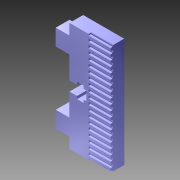
# Autodesk Inventor part: brida correas eje y
Saved by Autodesk Inventor 2012 SP2 (Build 160219200, 219)
## iProperties
Created: 2014-07-08
Part Number: brida correas eje y
Material: Default
Document SubType Name: Modeling
Designer: Principal
Density: 1 g/cm^3
Author: Principal
Autodesk Inventor part; units mm, degrees
ref_plane "YZ Plane" through (0, 0, 0) normal (1, 0, 0) x (0, 1, 0)
ref_plane "XZ Plane" through (0, 0, 0) normal (0, 1, 0) x (-1, 0, 0)
ref_plane "XY Plane" through (0, 0, 0) normal (0, 0, 1) x (1, 0, 0)
sketch "Boceto1" plane through (0, 0, 0) normal (0, 0, 1) x (1, 0, 0)
  line L0 (0, 0) -> (15, 0)
  line L1 (15, 0) -> (15, -5)
  line L2 (15, -5) -> (0, -5)
  line L3 (0, -5) -> (0, 0)
  constraints: 8 end point
extrude "Extrusión1" add sketch "Boceto1" along normal blind 40
sketch "Boceto2" plane through (0, 0, 0) normal (0, 1, 0) x (1, 0, 0)
  line L0 (0, -40) -> (15, -40) projected
  line L1 (6.174, -21.75) -> (6.174, -18.25)
  line L2 (2.774, -22.75) -> (5.174, -22.75)
  line L3 (5.174, -17.25) -> (2.774, -17.25)
  line L4 (6.174, -18.25) -> (5.174, -18.25)
  line L5 (2.774, -18.25) -> (0, -18.25)
  line L6 (2.774, -17.25) -> (2.774, -18.25)
  line L7 (2.774, -21.75) -> (2.774, -22.75)
  line L8 (5.174, -22.75) -> (5.174, -21.75)
  line L9 (5.174, -18.25) -> (5.174, -17.25)
  line L10 (0, -21.75) -> (2.774, -21.75)
  line L11 (5.174, -21.75) -> (6.174, -21.75)
  line L12 (0, -10) -> (-5, -10)
  line L13 (-5, -10) -> (-5, -4)
  line L14 (-5, -4) -> (0, -4)
  line L15 (0, -4) -> (0, -10)
  line L16 (0, -36) -> (-5, -36)
  line L17 (-5, -36) -> (-5, -30)
  line L18 (-5, -30) -> (0, -30)
  line L19 (0, -30) -> (0, -36)
  line L20 (0, 0) -> (0, -40) projected
  dimension "d7" = 3.5
  dimension "d8" = 2.4
  dimension "d12" = 18.25
  dimension "d14" = 6
  dimension "d15" = 5
  dimension "d16" = 5
  dimension "d17" = 6
  dimension "d18" = 4
  dimension "d19" = 20
  constraints: 38 end point, 2 point on line
  measures "d7" distance of L1.end L1.start
  measures "d8" distance of L3.end L3.start
  measures "d12" distance from line of L0 L1.start
  measures "d14" distance between parallel lines of L18 L16
  measures "d15" distance between parallel lines of L19 L17
  measures "d16" distance between parallel lines of L15 L13
  measures "d17" distance between parallel lines of L12 L14
  measures "d18" distance between parallel lines of L0 L16
  measures "d19" distance between parallel lines of L12 L18
extrude "Extrusión3" cut sketch "Boceto2" against normal through all
sketch "Boceto3" plane through (0, 0, 0) normal (0, 1, 0) x (1, 0, 0)
  line L0 (2.774, -21.75) -> (0, -21.75) projected
  line L1 (0, -18.25) -> (2.774, -18.25) projected
  line L2 (-5, -10) -> (-5, -4)
  line L3 (-5, -36) -> (-5, -30)
  line L4 (-5, -36) -> (0, -36)
  line L5 (-5, -30) -> (0, -30)
  line L6 (-5, -4) -> (0, -4)
  line L7 (-5, -10) -> (0, -10)
  line L8 (0, -4) -> (0, -10)
  line L9 (0, -30) -> (0, -36)
  constraints: 18 end point
extrude "Extrusión4" add sketch "Boceto3" against normal blind 5
sketch "Boceto4" plane through (15, -5, 0) normal (1, 0, 0) x (0, 0, -1)
  arc A0 (-37.4947, 0.496) -> (-38.4947, 0.496) centre (-37.9947, 0.496) ccw
  line L0 (-38.4947, 0.496) -> (-38.4947, -0.004)
  line L1 (-37.4947, 0.496) -> (-37.4947, -0.004)
  line L2 (-39.4947, 0.496) -> (-39.4947, -0.004)
  arc A1 (-39.4947, 0.496) -> (-39.9947, 0.996) centre (-39.9947, 0.496) ccw
  arc A2 (-35.9947, 0.996) -> (-36.4947, 0.496) centre (-35.9947, 0.496) ccw
  line L3 (-36.4947, -0.004) -> (-36.4947, 0.496)
  arc A3 (-33.4947, 0.496) -> (-34.4947, 0.496) centre (-33.9947, 0.496) ccw
  line L4 (-34.4947, 0.496) -> (-34.4947, -0.004)
  line L5 (-33.4947, 0.496) -> (-33.4947, -0.004)
  line L6 (-35.4947, 0.496) -> (-35.4947, -0.004)
  arc A4 (-35.4947, 0.496) -> (-35.9947, 0.996) centre (-35.9947, 0.496) ccw
  arc A5 (-31.9947, 0.996) -> (-32.4947, 0.496) centre (-31.9947, 0.496) ccw
  line L7 (-32.4947, -0.004) -> (-32.4947, 0.496)
  arc A6 (-29.4947, 0.496) -> (-30.4947, 0.496) centre (-29.9947, 0.496) ccw
  line L8 (-30.4947, 0.496) -> (-30.4947, -0.004)
  line L9 (-29.4947, 0.496) -> (-29.4947, -0.004)
  line L10 (-31.4947, 0.496) -> (-31.4947, -0.004)
  arc A7 (-31.4947, 0.496) -> (-31.9947, 0.996) centre (-31.9947, 0.496) ccw
  arc A8 (-27.9947, 0.996) -> (-28.4947, 0.496) centre (-27.9947, 0.496) ccw
  line L11 (-28.4947, -0.004) -> (-28.4947, 0.496)
  line L12 (-26.4947, 0.496) -> (-26.4947, -0.004)
  line L13 (-25.4947, 0.496) -> (-25.4947, -0.004)
  line L14 (-27.4947, 0.496) -> (-27.4947, -0.004)
  line L15 (-24.4947, -0.004) -> (-24.4947, 0.496)
  arc A9 (-23.9947, 0.996) -> (-24.4947, 0.496) centre (-23.9947, 0.496) ccw
  arc A10 (-25.4947, 0.496) -> (-26.4947, 0.496) centre (-25.9947, 0.496) ccw
  arc A11 (-27.4947, 0.496) -> (-27.9947, 0.996) centre (-27.9947, 0.496) ccw
  arc A12 (-21.4947, 0.496) -> (-22.4947, 0.496) centre (-21.9947, 0.496) ccw
  line L16 (-22.4947, 0.496) -> (-22.4947, -0.004)
  line L17 (-21.4947, 0.496) -> (-21.4947, -0.004)
  line L18 (-23.4947, 0.496) -> (-23.4947, -0.004)
  arc A13 (-23.4947, 0.496) -> (-23.9947, 0.996) centre (-23.9947, 0.496) ccw
  arc A14 (-19.9947, 0.996) -> (-20.4947, 0.496) centre (-19.9947, 0.496) ccw
  line L19 (-20.4947, -0.004) -> (-20.4947, 0.496)
  line L20 (-18.4947, 0.496) -> (-18.4947, -0.004)
  line L21 (-17.4947, 0.496) -> (-17.4947, -0.004)
  line L22 (-19.4947, 0.496) -> (-19.4947, -0.004)
  line L23 (-16.4947, -0.004) -> (-16.4947, 0.496)
  arc A15 (-15.9947, 0.996) -> (-16.4947, 0.496) centre (-15.9947, 0.496) ccw
  arc A16 (-17.4947, 0.496) -> (-18.4947, 0.496) centre (-17.9947, 0.496) ccw
  arc A17 (-19.4947, 0.496) -> (-19.9947, 0.996) centre (-19.9947, 0.496) ccw
  arc A18 (-15.4947, 0.496) -> (-15.9947, 0.996) centre (-15.9947, 0.496) ccw
  line L24 (-14.4947, 0.496) -> (-14.4947, -0.004)
  arc A19 (-13.4947, 0.496) -> (-14.4947, 0.496) centre (-13.9947, 0.496) ccw
  line L25 (-13.4947, 0.496) -> (-13.4947, -0.004)
  line L26 (-12.4947, -0.004) -> (-12.4947, 0.496)
  arc A20 (-11.9947, 0.996) -> (-12.4947, 0.496) centre (-11.9947, 0.496) ccw
  arc A21 (-11.4947, 0.496) -> (-11.9947, 0.996) centre (-11.9947, 0.496) ccw
  line L27 (-11.4947, 0.496) -> (-11.4947, -0.004)
  line L28 (-15.4947, 0.496) -> (-15.4947, -0.004)
  line L29 (-10.4947, 0.496) -> (-10.4947, -0.004)
  arc A22 (-9.4947, 0.496) -> (-10.4947, 0.496) centre (-9.9947, 0.496) ccw
  line L30 (-9.4947, 0.496) -> (-9.4947, -0.004)
  line L31 (-8.4947, -0.004) -> (-8.4947, 0.496)
  arc A23 (-7.9947, 0.996) -> (-8.4947, 0.496) centre (-7.9947, 0.496) ccw
  arc A24 (0.0053, 0.996) -> (-0.4947, 0.496) centre (0.0053, 0.496) ccw
  line L32 (-0.4947, -0.004) -> (-0.4947, 0.496)
  arc A25 (-5.4947, 0.496) -> (-6.4947, 0.496) centre (-5.9947, 0.496) ccw
  line L33 (-6.4947, 0.496) -> (-6.4947, -0.004)
  line L34 (-7.4947, 0.496) -> (-7.4947, -0.004)
  arc A26 (-7.4947, 0.496) -> (-7.9947, 0.996) centre (-7.9947, 0.496) ccw
  line L35 (-5.4947, 0.496) -> (-5.4947, -0.004)
  line L36 (-4.4947, -0.004) -> (-4.4947, 0.496)
  arc A27 (-3.9947, 0.996) -> (-4.4947, 0.496) centre (-3.9947, 0.496) ccw
  arc A28 (-3.4947, 0.496) -> (-3.9947, 0.996) centre (-3.9947, 0.496) ccw
  line L37 (-3.4947, 0.496) -> (-3.4947, -0.004)
  line L38 (-2.4947, 0.496) -> (-2.4947, -0.004)
  arc A29 (-1.4947, 0.496) -> (-2.4947, 0.496) centre (-1.9947, 0.496) ccw
  line L39 (-1.4947, 0.496) -> (-1.4947, -0.004)
  line L40 (-0.4947, -0.004) -> (0.0053, -0.004)
  line L41 (-2.4947, -0.004) -> (-1.4947, -0.004)
  line L42 (-4.4947, -0.004) -> (-3.4947, -0.004)
  line L43 (-6.4947, -0.004) -> (-5.4947, -0.004)
  line L44 (-8.4947, -0.004) -> (-7.4947, -0.004)
  line L45 (-10.4947, -0.004) -> (-9.4947, -0.004)
  line L46 (-12.4947, -0.004) -> (-11.4947, -0.004)
  line L47 (-14.4947, -0.004) -> (-13.4947, -0.004)
  line L48 (-16.4947, -0.004) -> (-15.4947, -0.004)
  line L49 (-18.4947, -0.004) -> (-17.4947, -0.004)
  line L50 (-24.4947, -0.004) -> (-23.4947, -0.004)
  line L51 (-22.4947, -0.004) -> (-21.4947, -0.004)
  line L52 (-20.4947, -0.004) -> (-19.4947, -0.004)
  line L53 (-26.4947, -0.004) -> (-25.4947, -0.004)
  line L54 (-28.4947, -0.004) -> (-27.4947, -0.004)
  line L55 (-30.4947, -0.004) -> (-29.4947, -0.004)
  line L56 (-32.4947, -0.004) -> (-31.4947, -0.004)
  line L57 (-34.4947, -0.004) -> (-33.4947, -0.004)
  line L58 (-36.4947, -0.004) -> (-35.4947, -0.004)
  line L59 (-39.9947, -0.004) -> (-39.4947, -0.004)
  line L60 (-38.4947, -0.004) -> (-37.4947, -0.004)
  line L61 (0.0053, -0.004) -> (0.0053, 0.996)
  line L62 (-39.9947, -0.004) -> (-40.0154, -0.004)
  line L63 (-40.0154, -0.004) -> (-40.0154, 0.996)
  line L64 (-40.0154, 0.996) -> (-39.9947, 0.996)
  point P0 (-32.9947, 0.496)
  point P1 (-30.9947, 0.496)
  point P2 (-28.9947, 0.496)
  point P3 (-24.9947, 0.496)
  point P4 (-26.9947, 0.496)
  point P5 (-22.9947, 0.496)
  point P6 (-20.9947, 0.496)
  point P7 (-16.9947, 0.496)
  point P8 (-18.9947, 0.496)
  point P9 (-10.9947, 0.496)
  point P10 (-8.9947, 0.496)
  point P11 (-12.9947, 0.496)
  point P12 (-14.9947, 0.496)
  point P13 (-2.9947, 0.496)
  point P14 (-0.9947, 0.496)
  point P15 (-4.9947, 0.496)
  point P16 (-6.9947, 0.496)
  dimension "d49" = 4
  dimension "d50" = 8
  dimension "d51" = 4
  constraints: 130 end point, 60 point on circle, 30 centre point
  measures "d49" distance of L16.end L20.end
  measures "d50" distance of L18.start L28.start
  measures "d51" distance of L33.end L38.end
extrude "Extrusión5" cut sketch "Boceto4" against normal blind 8
